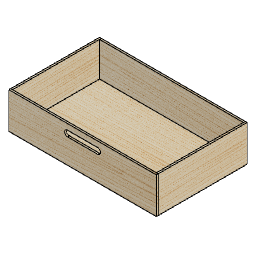
model (Autodesk Fusion 360 design; units mm, degrees)
Autodesk Fusion 360 part; units mm, degrees
sketch "Sketch1" plane through (0, 0, 0) normal (0, 1, 0) x (1, 0, 0) in component "box"
  line L0 (0, 0) -> (488, 0)
  line L1 (488, 0) -> (488, -119.5)
  line L2 (488, -119.5) -> (0, -119.5)
  line L3 (0, -119.5) -> (0, 0)
  line L4 (194, -100.45) -> (294, -100.45)
  arc A0 (294, -100.45) -> (294, -81.4) centre (294, -90.925) ccw
  line L5 (294, -81.4) -> (194, -81.4)
  arc A1 (194, -81.4) -> (194, -100.45) centre (194, -90.925) ccw
  line L6 (294, -90.925) -> (488, -90.925) construction
  line L7 (194, -90.925) -> (0, -90.925) construction
  dimension "d9" = 119.5
  dimension "d10" = 488
  dimension "d11" = 19.05
  dimension "d12" = 100
  dimension "d13" = 19.05
  constraint horizontal L0
  constraint vertical L1
  constraint horizontal L2
  constraint vertical L3
  constraint coincident L0.start L3.end
  constraint parallel L2 L4
  constraint tangent L4 A0
  constraint tangent A0 L5
  constraint parallel L4 L5
  constraint tangent L5 A1
  constraint tangent L4 A1
  constraint coincident A0.centre L6.start
  constraint coincident L1 L6.end
  constraint perpendicular L1 L6
  constraint coincident A1.centre L7.start
  constraint coincident L3 L7.end
  constraint perpendicular L3 L7
  constraint equal L6 L7
  measures "d9" distance of L0.start L2.end
  measures "d10" distance of L0.start L0.end
  measures "d11" distance of L4 L5
  measures "d12" distance of A0.end L5.end
  measures "d13" distance of L2 L4.start
extrude "Extrude1" add sketch "Sketch1" along normal blind 6 makes body 1 in component "box"
sketch "Sketch2" plane through (488, 0, 0) normal (1, 0, 0) x (0, 1, 0) in component "box"
  line L0 (0, 119.5) -> (0, 0)
  line L1 (0, 0) -> (6, 0)
  line L2 (6, 0) -> (6, 119.5)
  line L3 (6, 119.5) -> (0, 119.5)
  line L4 (6, 0) -> (300, 0)
  line L5 (300, 0) -> (300, 119.5)
  line L6 (300, 119.5) -> (6, 119.5)
  line L7 (6, 119.5) -> (6, 0)
  dimension "d16" = 294
  dimension "d17" = 119.5
  constraint horizontal L4
  constraint vertical L5
  constraint horizontal L6
  constraint vertical L7
  constraint coincident L1.end L2.start
  measures "d16" distance of L1.end L4.end
  measures "d17" distance of L1.end L2.end
extrude "Extrude2" add sketch "Sketch2" against normal blind 6 separate body contours L2 L4 L5 L6 L7 makes body 2 in component "box"
extrude "Extrude3" add sketch "Sketch2" along normal blind -488 and the other way blind 482 separate body contours L2 L4 L5 L6 L7 makes body 3 in component "box"
sketch "Sketch3" plane through (0, 300, 0) normal (0, 1, 0) x (-1, 0, 0) in component "box"
  line L0 (-6, 119.5) -> (-6, 0)
  line L1 (-6, 0) -> (0, 0)
  line L2 (0, 0) -> (0, 119.5)
  line L3 (0, 119.5) -> (-6, 119.5)
  line L4 (0, 0) -> (-6, 0) construction
  line L5 (-6, 0) -> (-482, 0)
  line L6 (-482, 0) -> (-482, 119.5)
  line L7 (-482, 119.5) -> (-6, 119.5)
  line L8 (-6, 119.5) -> (-6, 0)
  dimension "d24" = 6
  dimension "d25" = 476
  dimension "d26" = 119.5
  constraint coincident L1.end L2.start
  constraint perpendicular L2 L4
  constraint horizontal L5
  constraint vertical L6
  constraint horizontal L7
  constraint vertical L8
  constraint coincident L0.end L1.start
  measures "d24" distance of L1.end L0.end
  measures "d25" distance of L0.end L5.end
  measures "d26" distance of L0.end L0.start
extrude "Extrude4" add sketch "Sketch3" against normal blind 6 separate body contours L0 L5 L6 L7 L8 makes body 4 in component "box"
sketch "Sketch4" plane through (0, 0, 0) normal (0, 0, 1) x (1, 0, 0) in component "box"
  line L0 (0, 0) -> (6, 6) construction
  line L1 (0, 0) -> (9.1956, 0) construction
  line L2 (6, 6) -> (482, 6)
  line L3 (482, 6) -> (482, 294)
  line L4 (482, 294) -> (6, 294)
  line L5 (6, 294) -> (6, 6)
  dimension "d29" = 45
  dimension "d30" = 6
  dimension "d31" = 476
  dimension "d32" = 288
  constraint horizontal L1
  constraint coincident L0.start L1.start
  constraint horizontal L2
  constraint vertical L3
  constraint horizontal L4
  constraint vertical L5
  measures "d29" angle of L0 L1
  measures "d30" horizontal distance of L0.start L0.end
  measures "d31" distance of L3.end L4.end
  measures "d32" distance of L2.end L3.end
extrude "Extrude5" add sketch "Sketch4" along normal blind 6 separate body makes body 5 in component "box"
sketch "Sketch5" plane through (0, 0, 0) normal (0, 0, 1) x (1, 0, 0) in component "box"
  line L0 (75, 75) -> (115, 75)
  line L1 (115, 75) -> (115, 300)
  line L2 (115, 300) -> (75, 300)
  line L3 (75, 300) -> (75, 75)
  line L4 (413, 300) -> (373, 300)
  line L5 (373, 300) -> (373, 75)
  line L6 (373, 75) -> (413, 75)
  line L7 (413, 75) -> (413, 300)
  line L8 (0, 0) -> (488, 0) construction
  dimension "d35" = 40
  dimension "d36" = 225
  dimension "d37" = 40
  dimension "d38" = 225
  dimension "d40" = 75
  dimension "d41" = 75
  dimension "d42" = 488
  dimension "d43" = 75
  dimension "d44" = 75
  constraint horizontal L0
  constraint vertical L1
  constraint horizontal L2
  constraint vertical L3
  constraint horizontal L4
  constraint vertical L5
  constraint horizontal L6
  constraint vertical L7
  constraint coincident L8.start origin
  constraint horizontal L8
  measures "d35" distance of L0.start L0.end
  measures "d36" distance of L0.start L2.end
  measures "d37" distance of L4.start L4.end
  measures "d38" distance of L4.start L6.end
  measures "d40" distance of L8.start L3
  measures "d41" distance of L8.start L0
  measures "d42" distance of L8.start L8.end
  measures "d43" distance of L7 L8.end
  measures "d44" distance of L6 L8.end
extrude "Extrude6" add sketch "Sketch5" against normal blind 6 separate body makes body 6 at (88.3333, 225, 0) makes body 7 at (386.3333, 225, 0) in component "box"
component "box" placed x (1, 0, 0) y (0, 1, 0) z (0, 0, 1) at (0, 0, 0)
equation "thickness = 6 mm"
equation "width = 500 mm - ( 2 * thickness )"
equation "height = 131.5 mm - ( 2 * thickness )"
equation "depth = 300 mm"
equation "forstner = 1 in * 0.75"
equation "handle_width = 100 mm"
equation "skate_offset = depth / 4"
equation "d9 = height"
equation "d10 = width"
equation "d11 = forstner"
equation "d12 = handle_width"
equation "d13 = forstner"
equation "d14 = thickness"
equation "d16 = depth - thickness"
equation "d17 = height"
equation "d18 = -thickness"
equation "d20 = -width"
equation "d22 = width - thickness"
equation "d24 = thickness"
equation "d25 = width - ( 2 * thickness )"
equation "d26 = height"
equation "d27 = -thickness"
equation "d30 = thickness"
equation "d31 = width - ( 2 * thickness )"
equation "d32 = depth - ( 2 * thickness )"
equation "d33 = thickness"
equation "d35 = skate_width"
equation "d36 = depth - skate_offset"
equation "d37 = skate_width"
equation "d38 = depth - skate_offset"
equation "skate_width = 40 mm"
equation "d40 = skate_offset"
equation "d41 = skate_offset"
equation "d42 = width"
equation "d43 = skate_offset"
equation "d44 = skate_offset"
equation "d45 = -thickness"
